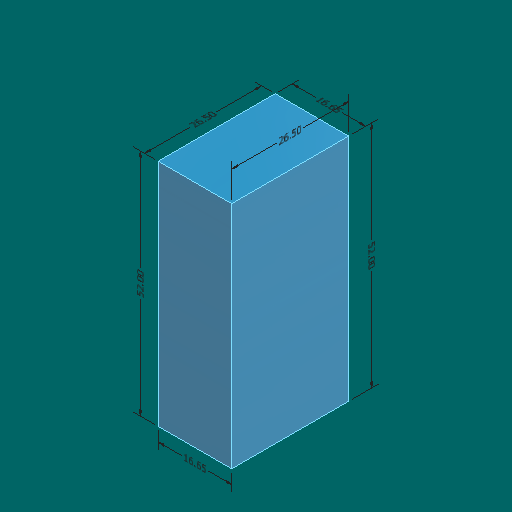
# Autodesk Inventor part: 9V_Battery
Saved by Autodesk Inventor 2025.2 (Build 292293000, 293)
## iProperties
Created: 2025-04-19
Part Number: 9V_Battery
Material: Generic
Document SubType Name: Modeling
Designer: Matt Caldwell
Density: 1 g/cm^3
Appearance: Default
Author: Matt Caldwell
Autodesk Inventor part; units mm, degrees
ref_plane "YZ Plane" through (0, 0, 0) normal (1, 0, 0) x (0, 1, 0)
ref_plane "XZ Plane" through (0, 0, 0) normal (0, 1, 0) x (-1, 0, 0)
ref_plane "XY Plane" through (0, 0, 0) normal (0, 0, 1) x (1, 0, 0)
sketch "Sketch1" plane through (0, 0, 0) normal (0, 1, 0) x (-1, 0, 0)
  line L0 (10.4115, 12.4771) -> (-6.2385, 12.4771)
  line L1 (-6.2385, 12.4771) -> (-6.2385, -14.0229)
  line L2 (-6.2385, -14.0229) -> (10.4115, -14.0229)
  line L3 (10.4115, -14.0229) -> (10.4115, 12.4771)
  dimension "d2" = 26.5
  dimension "d3" = 16.65
  constraints: 8 end point, 2 parallel, 1 horizontal, 1 perpendicular
  measures "d2" distance between parallel lines of L2 L0
  measures "d3" distance between parallel lines of L1 L3
extrude "Extrusion1" add sketch "Sketch1" along normal blind 52
body "Solid1"
